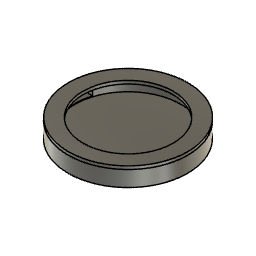
Microphone Holder Prototype v2 (Autodesk Fusion 360 design; units mm, degrees)
Autodesk Fusion 360 part; units mm, degrees
sketch "Sketch1" plane through (0, 0, 0) normal (0, 0, 1) x (1, 0, 0)
  circle A0 centre (0, 0) radius 381
  dimension "d1" = 762
  constraint coincident A0.centre origin
  measures "d1" diameter of A0
extrude "Extrude1" add sketch "Sketch1" along normal blind 100 makes body 1
hole "Hole1" at (0, 0, 100) direction (0, 0, -1) diameter 680 depth 80 tip angle 180 bodies 1
sketch "Sketch2" plane through (0, 0, 0) normal (0, 0, 1) x (1, 0, 0)
  circle A0 centre (-1124.3178, 355.266) radius 381
  dimension "d7" = 762
  measures "d7" diameter of A0
extrude "Extrude2" add sketch "Sketch2" along normal blind 100 separate body makes body 2
extrude "Extrude3" cut 1 faces at (-1008.2271, 247.5495, 0) along direction (0, 0, 1) blind 80 on bodies 2 bodies 2
move_body "Move1" bodies 2 to x (1, 0, 0) y (0, 1, 0) z (0, 0, 1) at (1125, -355, 0)
move_body "Move2" bodies 2 to x (1, 0, 0) y (0, 1, 0) z (0, 0, 1) at (0, 0, 20)
hole "Hole2" at (0.6822, 0.266, 120) direction (0, 0, -1) diameter 575 depth 60 tip angle 180 bodies 2
sketch "Sketch3" plane through (0, 0, 0) normal (1, 0, 0) x (0, 1, 0)
  line L0 (-100, 100) -> (100, 100)
  line L1 (100, 100) -> (100, 25)
  line L2 (100, 25) -> (-100, 25)
  line L3 (-100, 25) -> (-100, 100)
  constraint horizontal L0
  constraint vertical L1
  constraint horizontal L2
  constraint vertical L3
extrude "Extrude4" cut sketch "Sketch3" against normal blind 2000 bodies 1
hole "Hole3" [suppressed]
